Autodesk Fusion 360 part; units mm, degrees
(part 3 of 8)
  spline S13 degree 5 poles (-0.7278, 10.3745) (-0.7298, 10.3716) (-0.7338, 10.3659) (-0.7399, 10.3573) (-0.7479, 10.3459) (-0.7578, 10.3316) (-0.7677, 10.3173) (-0.7776, 10.303) (-0.7874, 10.2887) (-0.7971, 10.2744) (-0.8067, 10.2601) (-0.8163, 10.2458) (-0.8259, 10.2316) (-0.8354, 10.2173) (-0.8448, 10.203) (-0.8542, 10.1888) (-0.8635, 10.1745) (-0.8727, 10.1603) (-0.8819, 10.1461) (-0.891, 10.1318) (-0.9001, 10.1176) (-0.9091, 10.1034) (-0.918, 10.0892) (-0.9269, 10.075) (-0.9357, 10.0608) (-0.9445, 10.0467) (-0.9532, 10.0325) (-0.9619, 10.0184) (-0.9705, 10.0042) (-0.979, 9.9901) (-0.9875, 9.976) (-0.9959, 9.9619) (-1.0042, 9.9478) (-1.0125, 9.9337) (-1.0207, 9.9196) (-1.0289, 9.9056) (-1.037, 9.8915) (-1.0451, 9.8775) (-1.0531, 9.8635) (-1.061, 9.8494) (-1.0689, 9.8355) (-1.0767, 9.8215) (-1.0845, 9.8075) (-1.0922, 9.7936) (-1.0998, 9.7796) (-1.1074, 9.7657) (-1.1149, 9.7518) (-1.1224, 9.7379) (-1.1298, 9.7241) (-1.1371, 9.7102) (-1.1444, 9.6964) (-1.1516, 9.6825) (-1.1588, 9.6687) (-1.1659, 9.655) (-1.1729, 9.6412) (-1.1799, 9.6275) (-1.1868, 9.6137) (-1.1937, 9.6) (-1.2005, 9.5863) (-1.2073, 9.5727) (-1.214, 9.559) (-1.2206, 9.5454) (-1.2272, 9.5318) (-1.2337, 9.5182) (-1.2401, 9.5047) (-1.2465, 9.4911) (-1.2529, 9.4776) (-1.2592, 9.4641) (-1.2654, 9.4507) (-1.2716, 9.4372) (-1.2777, 9.4238) (-1.2837, 9.4104) (-1.2897, 9.397) (-1.2957, 9.3837) (-1.3015, 9.3704) (-1.3074, 9.3571) (-1.3131, 9.3438) (-1.3188, 9.3305) (-1.3245, 9.3173) (-1.3301, 9.3041) (-1.3356, 9.291) (-1.3411, 9.2778) (-1.3465, 9.2647) (-1.3518, 9.2517) (-1.3571, 9.2386) (-1.3624, 9.2256) (-1.3676, 9.2126) (-1.3727, 9.1997) (-1.3778, 9.1867) (-1.3828, 9.1738) (-1.3877, 9.161) (-1.3927, 9.1481) (-1.3975, 9.1353) (-1.4023, 9.1226) (-1.407, 9.1098) (-1.4117, 9.0971) (-1.4163, 9.0845) (-1.4209, 9.0718) (-1.4254, 9.0593) (-1.4299, 9.0467) (-1.4343, 9.0342) (-1.4386, 9.0217) (-1.4429, 9.0092) (-1.4471, 8.9968) (-1.4513, 8.9844) (-1.4554, 8.9721) (-1.4595, 8.9598) (-1.4635, 8.9475) (-1.4675, 8.9353) (-1.4714, 8.9231) (-1.4752, 8.9109) (-1.479, 8.8988) (-1.4828, 8.8868) (-1.4865, 8.8747) (-1.4901, 8.8628) (-1.4937, 8.8508) (-1.4972, 8.8389) (-1.5007, 8.8271) (-1.5041, 8.8153) (-1.5075, 8.8035) (-1.5108, 8.7918) (-1.514, 8.7801) (-1.5173, 8.7684) (-1.5204, 8.7569) (-1.5235, 8.7453) (-1.5266, 8.7338) (-1.5296, 8.7224) (-1.5325, 8.711) (-1.5354, 8.6996) (-1.5383, 8.6883) (-1.5411, 8.6771) (-1.5438, 8.6659) (-1.5465, 8.6547) (-1.5492, 8.6436) (-1.5517, 8.6325) (-1.5543, 8.6215) (-1.5568, 8.6106) (-1.5592, 8.5997) (-1.5616, 8.5889) (-1.564, 8.5781) (-1.5663, 8.5673) (-1.5685, 8.5567) (-1.5707, 8.546) (-1.5729, 8.5355) (-1.575, 8.525) (-1.577, 8.5145) (-1.5791, 8.5041) (-1.581, 8.4938) (-1.5829, 8.4835) (-1.5848, 8.4733) (-1.5866, 8.4631) (-1.5884, 8.453) (-1.5901, 8.443) (-1.5918, 8.433) (-1.5935, 8.4231) (-1.5951, 8.4132) (-1.5966, 8.4035) (-1.5981, 8.3937) (-1.5996, 8.3841) (-1.601, 8.3745) (-1.6024, 8.365) (-1.6037, 8.3555) (-1.605, 8.3461) (-1.6062, 8.3368) (-1.6074, 8.3276) (-1.6086, 8.3184) (-1.6097, 8.3093) (-1.6108, 8.3002) (-1.6118, 8.2913) (-1.6128, 8.2824) (-1.6138, 8.2735) (-1.6147, 8.2648) (-1.6156, 8.2561) (-1.6164, 8.2475) (-1.6172, 8.239) (-1.618, 8.2306) (-1.6187, 8.2222) (-1.6194, 8.2139) (-1.6201, 8.2057) (-1.6207, 8.1976) (-1.6213, 8.1895) (-1.6218, 8.1815) (-1.6223, 8.1737) (-1.6228, 8.1658) (-1.6233, 8.1581) (-1.6237, 8.1505) (-1.6241, 8.143) (-1.6244, 8.1355) (-1.6247, 8.1281) (-1.625, 8.1208) (-1.6253, 8.1136) (-1.6255, 8.1065) (-1.6257, 8.0995) (-1.6258, 8.0926) (-1.626, 8.0858) (-1.6261, 8.079) (-1.6262, 8.0724) (-1.6262, 8.0659) (-1.6263, 8.0594) (-1.6263, 8.0531) (-1.6262, 8.0468) (-1.6262, 8.0407) (-1.6261, 8.0346) (-1.626, 8.0287) (-1.6259, 8.0229) (-1.6258, 8.0171) (-1.6257, 8.0115) (-1.6255, 8.006) (-1.6253, 8.0006) (-1.6251, 7.9953) (-1.6249, 7.9901) (-1.6246, 7.985) (-1.6244, 7.9801) (-1.6241, 7.9752) (-1.6238, 7.9705) (-1.6235, 7.9659) (-1.6232, 7.9614) (-1.6229, 7.957) (-1.6226, 7.9528) (-1.6223, 7.9487) (-1.6219, 7.9447) (-1.6216, 7.9408) (-1.6212, 7.9371) (-1.6209, 7.9334) (-1.6205, 7.93) (-1.6202, 7.9266) (-1.6198, 7.9234) (-1.6195, 7.9204) (-1.6191, 7.9174) (-1.6188, 7.9146) (-1.6184, 7.912) (-1.6181, 7.9095) (-1.6178, 7.9072) (-1.6175, 7.905) (-1.6172, 7.9029) (-1.6169, 7.9011) (-1.6166, 7.8993) (-1.6164, 7.8978) (-1.6161, 7.8964) (-1.6159, 7.8951) (-1.6157, 7.8941) (-1.6156, 7.8933) (-1.6155, 7.8929) (-1.6155, 7.8926) (-1.6154, 7.8925) knots -1 -1 -1 -1 -1 -1 -0.99583333 -0.99166667 -0.9875 -0.98333333 -0.97916667 -0.975 -0.97083333 -0.96666667 -0.9625 -0.95833333 -0.95416667 -0.95 -0.94583333 -0.94166667 -0.9375 -0.93333333 -0.92916667 -0.925 -0.92083333 -0.91666667 -0.9125 -0.90833333 -0.90416667 -0.9 -0.89583333 -0.89166667 -0.8875 -0.88333333 -0.87916667 -0.875 -0.87083333 -0.86666667 -0.8625 -0.85833333 -0.85416667 -0.85 -0.84583333 -0.84166667 -0.8375 -0.83333333 -0.82916667 -0.825 -0.82083333 -0.81666667 -0.8125 -0.80833333 -0.80416667 -0.8 -0.79583333 -0.79166667 -0.7875 -0.78333333 -0.77916667 -0.775 -0.77083333 -0.76666667 -0.7625 -0.75833333 -0.75416667 -0.75 -0.74583333 -0.74166667 -0.7375 -0.73333333 -0.72916667 -0.725 -0.72083333 -0.71666667 -0.7125 -0.70833333 -0.70416667 -0.7 -0.69583333 -0.69166667 -0.6875 -0.68333333 -0.67916667 -0.675 -0.67083333 -0.66666667 -0.6625 -0.65833333 -0.65416667 -0.65 -0.64583333 -0.64166667 -0.6375 -0.63333333 -0.62916667 -0.625 -0.62083333 -0.61666667 -0.6125 -0.60833333 -0.60416667 -0.6 -0.59583333 -0.59166667 -0.5875 -0.58333333 -0.57916667 -0.575 -0.57083333 -0.56666667 -0.5625 -0.55833333 -0.55416667 -0.55 -0.54583333 -0.54166667 -0.5375 -0.53333333 -0.52916667 -0.525 -0.52083333 -0.51666667 -0.5125 -0.50833333 -0.50416667 -0.5 -0.49583333 -0.49166667 -0.4875 -0.48333333 -0.47916667 -0.475 -0.47083333 -0.46666667 -0.4625 -0.45833333 -0.45416667 -0.45 -0.44583333 -0.44166667 -0.4375 -0.43333333 -0.42916667 -0.425 -0.42083333 -0.41666667 -0.4125 -0.40833333 -0.40416667 -0.4 -0.39583333 -0.39166667 -0.3875 -0.38333333 -0.37916667 -0.375 -0.37083333 -0.36666667 -0.3625 -0.35833333 -0.35416667 -0.35 -0.34583333 -0.34166667 -0.3375 -0.33333333 -0.32916667 -0.325 -0.32083333 -0.31666667 -0.3125 -0.30833333 -0.30416667 -0.3 -0.29583333 -0.29166667 -0.2875 -0.28333333 -0.27916667 -0.275 -0.27083333 -0.26666667 -0.2625 -0.25833333 -0.25416667 -0.25 -0.24583333 -0.24166667 -0.2375 -0.23333333 -0.22916667 -0.225 -0.22083333 -0.21666667 -0.2125 -0.20833333 -0.20416667 -0.2 -0.19583333 -0.19166667 -0.1875 -0.18333333 -0.17916667 -0.175 -0.17083333 -0.16666667 -0.1625 -0.15833333 -0.15416667 -0.15 -0.14583333 -0.14166667 -0.1375 -0.13333333 -0.12916667 -0.125 -0.12083333 -0.11666667 -0.1125 -0.10833333 -0.10416667 -0.1 -0.09583333 -0.09166667 -0.0875 -0.08333333 -0.07916667 -0.075 -0.07083333 -0.06666667 -0.0625 -0.05833333 -0.05416667 -0.05 -0.04583333 -0.04166667 -0.0375 -0.03333333 -0.02916667 -0.025 -0.02083333 -0.01666667 -0.0125 -0.00833333 -0.00416667 0 0 0 0 0 0
  line L26 (-1.6154, 7.8925) -> (-1.6152, 7.8914)
  line L27 (-1.6152, 7.8914) -> (-1.147, 5.6038)
  arc A14 (-1.147, 5.6038) -> (-3.1514, 4.7736) centre (0, 0) ccw
  line L28 (-3.1514, 4.7736) -> (-4.4379, 6.7222)
  line L29 (-4.4379, 6.7222) -> (-4.4385, 6.7231)
  spline S14 degree 5 poles (-4.4385, 6.7231) (-4.4386, 6.7232) (-4.4388, 6.7235) (-4.439, 6.7238) (-4.4394, 6.7244) (-4.4401, 6.7253) (-4.4408, 6.7263) (-4.4416, 6.7275) (-4.4425, 6.7288) (-4.4436, 6.7302) (-4.4447, 6.7317) (-4.4459, 6.7334) (-4.4473, 6.7352) (-4.4487, 6.737) (-4.4502, 6.739) (-4.4519, 6.7411) (-4.4536, 6.7434) (-4.4554, 6.7457) (-4.4573, 6.7481) (-4.4593, 6.7506) (-4.4614, 6.7532) (-4.4637, 6.7559) (-4.466, 6.7587) (-4.4684, 6.7616) (-4.4708, 6.7646) (-4.4734, 6.7677) (-4.4761, 6.7708) (-4.4789, 6.774) (-4.4818, 6.7774) (-4.4847, 6.7807) (-4.4878, 6.7842) (-4.4909, 6.7877) (-4.4942, 6.7914) (-4.4975, 6.7951) (-4.5009, 6.7988) (-4.5044, 6.8026) (-4.508, 6.8065) (-4.5117, 6.8105) (-4.5155, 6.8145) (-4.5194, 6.8186) (-4.5233, 6.8227) (-4.5274, 6.8269) (-4.5315, 6.8312) (-4.5357, 6.8355) (-4.54, 6.8399) (-4.5444, 6.8443) (-4.5489, 6.8488) (-4.5535, 6.8533) (-4.5582, 6.8579) (-4.5629, 6.8626) (-4.5678, 6.8672) (-4.5727, 6.872) (-4.5777, 6.8768) (-4.5828, 6.8816) (-4.588, 6.8864) (-4.5932, 6.8914) (-4.5986, 6.8963) (-4.604, 6.9013) (-4.6096, 6.9063) (-4.6152, 6.9114) (-4.6208, 6.9165) (-4.6266, 6.9216) (-4.6325, 6.9268) (-4.6384, 6.932) (-4.6444, 6.9373) (-4.6505, 6.9426) (-4.6567, 6.9479) (-4.663, 6.9532) (-4.6693, 6.9586) (-4.6758, 6.964) (-4.6823, 6.9694) (-4.6889, 6.9749) (-4.6956, 6.9804) (-4.7023, 6.9859) (-4.7092, 6.9914) (-4.7161, 6.997) (-4.7231, 7.0025) (-4.7301, 7.0082) (-4.7373, 7.0138) (-4.7445, 7.0194) (-4.7518, 7.0251) (-4.7592, 7.0308) (-4.7667, 7.0365) (-4.7743, 7.0422) (-4.7819, 7.048) (-4.7896, 7.0537) (-4.7974, 7.0595) (-4.8052, 7.0653) (-4.8132, 7.0711) (-4.8212, 7.0769) (-4.8293, 7.0828) (-4.8375, 7.0886) (-4.8457, 7.0945) (-4.854, 7.1004) (-4.8624, 7.1062) (-4.8709, 7.1121) (-4.8794, 7.118) (-4.8881, 7.1239) (-4.8968, 7.1299) (-4.9055, 7.1358) (-4.9144, 7.1417) (-4.9233, 7.1477) (-4.9323, 7.1536) (-4.9414, 7.1596) (-4.9505, 7.1655) (-4.9597, 7.1715) (-4.969, 7.1775) (-4.9784, 7.1834) (-4.9878, 7.1894) (-4.9973, 7.1954) (-5.0069, 7.2014) (-5.0165, 7.2074) (-5.0262, 7.2133) (-5.036, 7.2193) (-5.0459, 7.2253) (-5.0558, 7.2313) (-5.0658, 7.2373) (-5.0759, 7.2432) (-5.0861, 7.2492) (-5.0963, 7.2552) (-5.1066, 7.2612) (-5.1169, 7.2671) (-5.1274, 7.2731) (-5.1379, 7.279) (-5.1484, 7.285) (-5.1591, 7.2909) (-5.1698, 7.2969) (-5.1805, 7.3028) (-5.1914, 7.3087) (-5.2023, 7.3147) (-5.2133, 7.3206) (-5.2243, 7.3265) (-5.2354, 7.3324) (-5.2466, 7.3383) (-5.2578, 7.3441) (-5.2692, 7.35) (-5.2805, 7.3559) (-5.292, 7.3617) (-5.3035, 7.3675) (-5.3151, 7.3734) (-5.3267, 7.3792) (-5.3384, 7.385) (-5.3502, 7.3908) (-5.362, 7.3965) (-5.3739, 7.4023) (-5.3859, 7.408) (-5.3979, 7.4138) (-5.41, 7.4195) (-5.4222, 7.4252) (-5.4344, 7.4309) (-5.4467, 7.4366) (-5.4591, 7.4422) (-5.4715, 7.4478) (-5.484, 7.4535) (-5.4965, 7.4591) (-5.5091, 7.4647) (-5.5218, 7.4702) (-5.5345, 7.4758) (-5.5473, 7.4813) (-5.5601, 7.4868) (-5.5731, 7.4923) (-5.586, 7.4978) (-5.5991, 7.5033) (-5.6122, 7.5087) (-5.6253, 7.5141) (-5.6385, 7.5195) (-5.6518, 7.5249) (-5.6651, 7.5302) (-5.6785, 7.5356) (-5.692, 7.5409) (-5.7055, 7.5462) (-5.7191, 7.5514) (-5.7327, 7.5567) (-5.7464, 7.5619) (-5.7602, 7.5671) (-5.774, 7.5722) (-5.7878, 7.5774) (-5.8018, 7.5825) (-5.8158, 7.5876) (-5.8298, 7.5927) (-5.8439, 7.5977) (-5.8581, 7.6028) (-5.8723, 7.6077) (-5.8865, 7.6127) (-5.9009, 7.6177) (-5.9152, 7.6226) (-5.9297, 7.6275) (-5.9442, 7.6323) (-5.9587, 7.6372) (-5.9733, 7.642) (-5.988, 7.6467) (-6.0027, 7.6515) (-6.0175, 7.6562) (-6.0323, 7.6609) (-6.0472, 7.6656) (-6.0621, 7.6702) (-6.0771, 7.6748) (-6.0921, 7.6794) (-6.1072, 7.6839) (-6.1224, 7.6884) (-6.1376, 7.6929) (-6.1528, 7.6974) (-6.1681, 7.7018) (-6.1835, 7.7062) (-6.1989, 7.7105) (-6.2144, 7.7149) (-6.2299, 7.7192) (-6.2454, 7.7234) (-6.2611, 7.7276) (-6.2767, 7.7318) (-6.2925, 7.736) (-6.3082, 7.7401) (-6.324, 7.7442) (-6.3399, 7.7483) (-6.3558, 7.7523) (-6.3718, 7.7563) (-6.3878, 7.7603) (-6.4039, 7.7642) (-6.42, 7.7681) (-6.4362, 7.7719) (-6.4524, 7.7758) (-6.4687, 7.7796) (-6.485, 7.7833) (-6.5014, 7.787) (-6.5178, 7.7907) (-6.5343, 7.7943) (-6.5508, 7.7979) (-6.5673, 7.8015) (-6.5839, 7.805) (-6.6006, 7.8085) (-6.6173, 7.812) (-6.634, 7.8154) (-6.6508, 7.8188) (-6.6677, 7.8221) (-6.6845, 7.8254) (-6.7015, 7.8287) (-6.7185, 7.8319) (-6.7355, 7.8351) (-6.7525, 7.8383) (-6.7697, 7.8414) (-6.7868, 7.8445) (-6.8006, 7.8469) (-6.8109, 7.8487) (-6.8178, 7.8499) (-6.8213, 7.8505) knots 0 0 0 0 0 0 0.00416667 0.00833333 0.0125 0.01666667 0.02083333 0.025 0.02916667 0.03333333 0.0375 0.04166667 0.04583333 0.05 0.05416667 0.05833333 0.0625 0.06666667 0.07083333 0.075 0.07916667 0.08333333 0.0875 0.09166667 0.09583333 0.1 0.10416667 0.10833333 0.1125 0.11666667 0.12083333 0.125 0.12916667 0.13333333 0.1375 0.14166667 0.14583333 0.15 0.15416667 0.15833333 0.1625 0.16666667 0.17083333 0.175 0.17916667 0.18333333 0.1875 0.19166667 0.19583333 0.2 0.20416667 0.20833333 0.2125 0.21666667 0.22083333 0.225 0.22916667 0.23333333 0.2375 0.24166667 0.24583333 0.25 0.25416667 0.25833333 0.2625 0.26666667 0.27083333 0.275 0.27916667 0.28333333 0.2875 0.29166667 0.29583333 0.3 0.30416667 0.30833333 0.3125 0.31666667 0.32083333 0.325 0.32916667 0.33333333 0.3375 0.34166667 0.34583333 0.35 0.35416667 0.35833333 0.3625 0.36666667 0.37083333 0.375 0.37916667 0.38333333 0.3875 0.39166667 0.39583333 0.4 0.40416667 0.40833333 0.4125 0.41666667 0.42083333 0.425 0.42916667 0.43333333 0.4375 0.44166667 0.44583333 0.45 0.45416667 0.45833333 0.4625 0.46666667 0.47083333 0.475 0.47916667 0.48333333 0.4875 0.49166667 0.49583333 0.5 0.50416667 0.50833333 0.5125 0.51666667 0.52083333 0.525 0.52916667 0.53333333 0.5375 0.54166667 0.54583333 0.55 0.55416667 0.55833333 0.5625 0.56666667 0.57083333 0.575 0.57916667 0.58333333 0.5875 0.59166667 0.59583333 0.6 0.60416667 0.60833333 0.6125 0.61666667 0.62083333 0.625 0.62916667 0.63333333 0.6375 0.64166667 0.64583333 0.65 0.65416667 0.65833333 0.6625 0.66666667 0.67083333 0.675 0.67916667 0.68333333 0.6875 0.69166667 0.69583333 0.7 0.70416667 0.70833333 0.7125 0.71666667 0.72083333 0.725 0.72916667 0.73333333 0.7375 0.74166667 0.74583333 0.75 0.75416667 0.75833333 0.7625 0.76666667 0.77083333 0.775 0.77916667 0.78333333 0.7875 0.79166667 0.79583333 0.8 0.80416667 0.80833333 0.8125 0.81666667 0.82083333 0.825 0.82916667 0.83333333 0.8375 0.84166667 0.84583333 0.85 0.85416667 0.85833333 0.8625 0.86666667 0.87083333 0.875 0.87916667 0.88333333 0.8875 0.89166667 0.89583333 0.9 0.90416667 0.90833333 0.9125 0.91666667 0.92083333 0.925 0.92916667 0.93333333 0.9375 0.94166667 0.94583333 0.95 0.95416667 0.95833333 0.9625 0.96666667 0.97083333 0.975 0.97916667 0.98333333 0.9875 0.99166667 0.99583333 1 1 1 1 1 1
  arc A15 (-6.8213, 7.8505) -> (-7.8505, 6.8213) centre (0, 0) ccw
  spline S15 degree 5 poles (-7.8505, 6.8213) (-7.8499, 6.8178) (-7.8487, 6.8109) (-7.8469, 6.8006) (-7.8445, 6.7868) (-7.8414, 6.7697) (-7.8383, 6.7525) (-7.8351, 6.7355) (-7.8319, 6.7185) (-7.8287, 6.7015) (-7.8254, 6.6845) (-7.8221, 6.6677) (-7.8188, 6.6508) (-7.8154, 6.634) (-7.812, 6.6173) (-7.8085, 6.6006) (-7.805, 6.5839) (-7.8015, 6.5673) (-7.7979, 6.5508) (-7.7943, 6.5343) (-7.7907, 6.5178) (-7.787, 6.5014) (-7.7833, 6.485) (-7.7796, 6.4687) (-7.7758, 6.4524) (-7.7719, 6.4362) (-7.7681, 6.42) (-7.7642, 6.4039) (-7.7603, 6.3878) (-7.7563, 6.3718) (-7.7523, 6.3558) (-7.7483, 6.3399) (-7.7442, 6.324) (-7.7401, 6.3082) (-7.736, 6.2925) (-7.7318, 6.2767) (-7.7276, 6.2611) (-7.7234, 6.2454) (-7.7192, 6.2299) (-7.7149, 6.2144) (-7.7105, 6.1989) (-7.7062, 6.1835) (-7.7018, 6.1681) (-7.6974, 6.1528) (-7.6929, 6.1376) (-7.6884, 6.1224) (-7.6839, 6.1072) (-7.6794, 6.0921) (-7.6748, 6.0771) (-7.6702, 6.0621) (-7.6656, 6.0472) (-7.6609, 6.0323) (-7.6562, 6.0175) (-7.6515, 6.0027) (-7.6467, 5.988) (-7.642, 5.9733) (-7.6372, 5.9587) (-7.6323, 5.9442) (-7.6275, 5.9297) (-7.6226, 5.9152) (-7.6177, 5.9009) (-7.6127, 5.8865) (-7.6077, 5.8723) (-7.6028, 5.8581) (-7.5977, 5.8439) (-7.5927, 5.8298) (-7.5876, 5.8158) (-7.5825, 5.8018) (-7.5774, 5.7878) (-7.5722, 5.774) (-7.5671, 5.7602) (-7.5619, 5.7464) (-7.5567, 5.7327) (-7.5514, 5.7191) (-7.5462, 5.7055) (-7.5409, 5.692) (-7.5356, 5.6785) (-7.5302, 5.6651) (-7.5249, 5.6518) (-7.5195, 5.6385) (-7.5141, 5.6253) (-7.5087, 5.6122) (-7.5033, 5.5991) (-7.4978, 5.586) (-7.4923, 5.5731) (-7.4868, 5.5601) (-7.4813, 5.5473) (-7.4758, 5.5345) (-7.4702, 5.5218) (-7.4647, 5.5091) (-7.4591, 5.4965) (-7.4535, 5.484) (-7.4478, 5.4715) (-7.4422, 5.4591) (-7.4366, 5.4467) (-7.4309, 5.4344) (-7.4252, 5.4222) (-7.4195, 5.41) (-7.4138, 5.3979) (-7.408, 5.3859) (-7.4023, 5.3739) (-7.3965, 5.362) (-7.3908, 5.3502) (-7.385, 5.3384) (-7.3792, 5.3267) (-7.3734, 5.3151) (-7.3675, 5.3035) (-7.3617, 5.292) (-7.3559, 5.2805) (-7.35, 5.2692) (-7.3441, 5.2578) (-7.3383, 5.2466) (-7.3324, 5.2354) (-7.3265, 5.2243) (-7.3206, 5.2133) (-7.3147, 5.2023) (-7.3087, 5.1914) (-7.3028, 5.1805) (-7.2969, 5.1698) (-7.2909, 5.1591) (-7.285, 5.1484) (-7.279, 5.1379) (-7.2731, 5.1274) (-7.2671, 5.1169) (-7.2612, 5.1066) (-7.2552, 5.0963) (-7.2492, 5.0861) (-7.2432, 5.0759) (-7.2373, 5.0658) (-7.2313, 5.0558) (-7.2253, 5.0459) (-7.2193, 5.036) (-7.2133, 5.0262) (-7.2074, 5.0165) (-7.2014, 5.0069) (-7.1954, 4.9973) (-7.1894, 4.9878) (-7.1834, 4.9784) (-7.1775, 4.969) (-7.1715, 4.9597) (-7.1655, 4.9505) (-7.1596, 4.9414) (-7.1536, 4.9323) (-7.1477, 4.9233) (-7.1417, 4.9144) (-7.1358, 4.9055) (-7.1299, 4.8968) (-7.1239, 4.8881) (-7.118, 4.8794) (-7.1121, 4.8709) (-7.1062, 4.8624) (-7.1004, 4.854) (-7.0945, 4.8457) (-7.0886, 4.8375) (-7.0828, 4.8293) (-7.0769, 4.8212) (-7.0711, 4.8132) (-7.0653, 4.8052) (-7.0595, 4.7974) (-7.0537, 4.7896) (-7.048, 4.7819) (-7.0422, 4.7743) (-7.0365, 4.7667) (-7.0308, 4.7592) (-7.0251, 4.7518) (-7.0194, 4.7445) (-7.0138, 4.7373) (-7.0082, 4.7301) (-7.0025, 4.7231) (-6.997, 4.7161) (-6.9914, 4.7092) (-6.9859, 4.7023) (-6.9804, 4.6956) (-6.9749, 4.6889) (-6.9694, 4.6823) (-6.964, 4.6758) (-6.9586, 4.6693) (-6.9532, 4.663) (-6.9479, 4.6567) (-6.9426, 4.6505) (-6.9373, 4.6444) (-6.932, 4.6384) (-6.9268, 4.6325) (-6.9216, 4.6266) (-6.9165, 4.6208) (-6.9114, 4.6152) (-6.9063, 4.6096) (-6.9013, 4.604) (-6.8963, 4.5986) (-6.8914, 4.5932) (-6.8864, 4.588) (-6.8816, 4.5828) (-6.8768, 4.5777) (-6.872, 4.5727) (-6.8672, 4.5678) (-6.8626, 4.5629) (-6.8579, 4.5582) (-6.8533, 4.5535) (-6.8488, 4.5489) (-6.8443, 4.5444) (-6.8399, 4.54) (-6.8355, 4.5357) (-6.8312, 4.5315) (-6.8269, 4.5274) (-6.8227, 4.5233) (-6.8186, 4.5194) (-6.8145, 4.5155) (-6.8105, 4.5117) (-6.8065, 4.508) (-6.8026, 4.5044) (-6.7988, 4.5009) (-6.7951, 4.4975) (-6.7914, 4.4942) (-6.7877, 4.4909) (-6.7842, 4.4878) (-6.7807, 4.4847) (-6.7774, 4.4818) (-6.774, 4.4789) (-6.7708, 4.4761) (-6.7677, 4.4734) (-6.7646, 4.4708) (-6.7616, 4.4684) (-6.7587, 4.466) (-6.7559, 4.4637) (-6.7532, 4.4614) (-6.7506, 4.4593) (-6.7481, 4.4573) (-6.7457, 4.4554) (-6.7434, 4.4536) (-6.7411, 4.4519) (-6.739, 4.4502) (-6.737, 4.4487) (-6.7352, 4.4473) (-6.7334, 4.4459) (-6.7317, 4.4447) (-6.7302, 4.4436) (-6.7288, 4.4425) (-6.7275, 4.4416) (-6.7263, 4.4408) (-6.7253, 4.4401) (-6.7244, 4.4394) (-6.7238, 4.439) (-6.7235, 4.4388) (-6.7232, 4.4386) (-6.7231, 4.4385) knots -1 -1 -1 -1 -1 -1 -0.99583333 -0.99166667 -0.9875 -0.98333333 -0.97916667 -0.975 -0.97083333 -0.96666667 -0.9625 -0.95833333 -0.95416667 -0.95 -0.94583333 -0.94166667 -0.9375 -0.93333333 -0.92916667 -0.925 -0.92083333 -0.91666667 -0.9125 -0.90833333 -0.90416667 -0.9 -0.89583333 -0.89166667 -0.8875 -0.88333333 -0.87916667 -0.875 -0.87083333 -0.86666667 -0.8625 -0.85833333 -0.85416667 -0.85 -0.84583333 -0.84166667 -0.8375 -0.83333333 -0.82916667 -0.825 -0.82083333 -0.81666667 -0.8125 -0.80833333 -0.80416667 -0.8 -0.79583333 -0.79166667 -0.7875 -0.78333333 -0.77916667 -0.775 -0.77083333 -0.76666667 -0.7625 -0.75833333 -0.75416667 -0.75 -0.74583333 -0.74166667 -0.7375 -0.73333333 -0.72916667 -0.725 -0.72083333 -0.71666667 -0.7125 -0.70833333 -0.70416667 -0.7 -0.69583333 -0.69166667 -0.6875 -0.68333333 -0.67916667 -0.675 -0.67083333 -0.66666667 -0.6625 -0.65833333 -0.65416667 -0.65 -0.64583333 -0.64166667 -0.6375 -0.63333333 -0.62916667 -0.625 -0.62083333 -0.61666667 -0.6125 -0.60833333 -0.60416667 -0.6 -0.59583333 -0.59166667 -0.5875 -0.58333333 -0.57916667 -0.575 -0.57083333 -0.56666667 -0.5625 -0.55833333 -0.55416667 -0.55 -0.54583333 -0.54166667 -0.5375 -0.53333333 -0.52916667 -0.525 -0.52083333 -0.51666667 -0.5125 -0.50833333 -0.50416667 -0.5 -0.49583333 -0.49166667 -0.4875 -0.48333333 -0.47916667 -0.475 -0.47083333 -0.46666667 -0.4625 -0.45833333 -0.45416667 -0.45 -0.44583333 -0.44166667 -0.4375 -0.43333333 -0.42916667 -0.425 -0.42083333 -0.41666667 -0.4125 -0.40833333 -0.40416667 -0.4 -0.39583333 -0.39166667 -0.3875 -0.38333333 -0.37916667 -0.375 -0.37083333 -0.36666667 -0.3625 -0.35833333 -0.35416667 -0.35 -0.34583333 -0.34166667 -0.3375 -0.33333333 -0.32916667 -0.325 -0.32083333 -0.31666667 -0.3125 -0.30833333 -0.30416667 -0.3 -0.29583333 -0.29166667 -0.2875 -0.28333333 -0.27916667 -0.275 -0.27083333 -0.26666667 -0.2625 -0.25833333 -0.25416667 -0.25 -0.24583333 -0.24166667 -0.2375 -0.23333333 -0.22916667 -0.225 -0.22083333 -0.21666667 -0.2125 -0.20833333 -0.20416667 -0.2 -0.19583333 -0.19166667 -0.1875 -0.18333333 -0.17916667 -0.175 -0.17083333 -0.16666667 -0.1625 -0.15833333 -0.15416667 -0.15 -0.14583333 -0.14166667 -0.1375 -0.13333333 -0.12916667 -0.125 -0.12083333 -0.11666667 -0.1125 -0.10833333 -0.10416667 -0.1 -0.09583333 -0.09166667 -0.0875 -0.08333333 -0.07916667 -0.075 -0.07083333 -0.06666667 -0.0625 -0.05833333 -0.05416667 -0.05 -0.04583333 -0.04166667 -0.0375 -0.03333333 -0.02916667 -0.025 -0.02083333 -0.01666667 -0.0125 -0.00833333 -0.00416667 0 0 0 0 0 0
  line L30 (-6.7231, 4.4385) -> (-6.7222, 4.4379)
  line L31 (-6.7222, 4.4379) -> (-4.7736, 3.1514)
  circle A16 centre (0, 0) radius 2.9
  dimension "d7" = 5.8
  constraint concentric A0 A16
  measures "d7" diameter of A16
sketch "Sketch1 (2)" plane through (0, 0, 0) normal (0, 0, 1) x (1, 0, 0) in component "Component"
  spline S0 degree 5 poles (8.6134, -1.763) (8.6136, -1.763) (8.6139, -1.7631) (8.6144, -1.7632) (8.6152, -1.7633) (8.6164, -1.7635) (8.6178, -1.7638) (8.6193, -1.764) (8.6211, -1.7643) (8.6231, -1.7646) (8.6252, -1.7649) (8.6275, -1.7653) (8.6299, -1.7656) (8.6326, -1.766) (8.6354, -1.7664) (8.6383, -1.7667) (8.6414, -1.7671) (8.6447, -1.7675) (8.6482, -1.7679) (8.6518, -1.7683) (8.6555, -1.7687) (8.6594, -1.7691) (8.6634, -1.7695) (8.6676, -1.7698) (8.6719, -1.7702) (8.6764, -1.7706) (8.681, -1.7709) (8.6857, -1.7713) (8.6906, -1.7716) (8.6956, -1.772) (8.7007, -1.7723) (8.706, -1.7726) (8.7114, -1.7729) (8.7169, -1.7732) (8.7226, -1.7734) (8.7283, -1.7736) (8.7342, -1.7739) (8.7402, -1.7741) (8.7464, -1.7742) (8.7526, -1.7744) (8.759, -1.7745) (8.7655, -1.7746) (8.772, -1.7747) (8.7787, -1.7748) (8.7856, -1.7748) (8.7925, -1.7748) (8.7995, -1.7748) (8.8067, -1.7747) (8.8139, -1.7747) (8.8212, -1.7746) (8.8287, -1.7744) (8.8362, -1.7743) (8.8439, -1.7741) (8.8517, -1.7738) (8.8595, -1.7736) (8.8675, -1.7733) (8.8755, -1.7729) (8.8836, -1.7726) (8.8919, -1.7722) (8.9002, -1.7717) (8.9086, -1.7712) (8.9172, -1.7707) (8.9258, -1.7702) (8.9345, -1.7696) (8.9432, -1.769) (8.9521, -1.7683) (8.9611, -1.7676) (8.9701, -1.7669) (8.9792, -1.7661) (8.9885, -1.7653) (8.9978, -1.7644) (9.0071, -1.7635) (9.0166, -1.7625) (9.0261, -1.7615) (9.0358, -1.7605) (9.0455, -1.7594) (9.0552, -1.7583) (9.0651, -1.7571) (9.075, -1.7559) (9.0851, -1.7547) (9.0951, -1.7534) (9.1053, -1.752) (9.1155, -1.7506) (9.1258, -1.7492) (9.1362, -1.7477) (9.1467, -1.7462) (9.1572, -1.7446) (9.1678, -1.743) (9.1785, -1.7413) (9.1892, -1.7396) (9.2, -1.7378) (9.2109, -1.736) (9.2218, -1.7341) (9.2328, -1.7322) (9.2439, -1.7302) (9.255, -1.7282) (9.2662, -1.7261) (9.2774, -1.724) (9.2888, -1.7218) (9.3001, -1.7196) (9.3116, -1.7173) (9.3231, -1.7149) (9.3347, -1.7126) (9.3463, -1.7101) (9.358, -1.7076) (9.3697, -1.7051) (9.3815, -1.7025) (9.3934, -1.6998) (9.4053, -1.6971) (9.4173, -1.6944) (9.4293, -1.6916) (9.4414, -1.6887) (9.4535, -1.6858) (9.4657, -1.6828) (9.4779, -1.6798) (9.4902, -1.6767) (9.5026, -1.6736) (9.515, -1.6704) (9.5274, -1.6671) (9.5399, -1.6638) (9.5525, -1.6604) (9.5651, -1.657) (9.5777, -1.6536) (9.5904, -1.65) (9.6032, -1.6464) (9.616, -1.6428) (9.6288, -1.6391) (9.6417, -1.6353) (9.6546, -1.6315) (9.6676, -1.6276) (9.6806, -1.6237) (9.6937, -1.6197) (9.7068, -1.6156) (9.72, -1.6115) (9.7332, -1.6074) (9.7464, -1.6031) (9.7597, -1.5989) (9.773, -1.5945) (9.7864, -1.5901) (9.7998, -1.5857) (9.8132, -1.5811) (9.8267, -1.5766) (9.8403, -1.5719) (9.8538, -1.5672) (9.8674, -1.5625) (9.8811, -1.5576) (9.8948, -1.5528) (9.9085, -1.5478) (9.9222, -1.5428) (9.936, -1.5378) (9.9498, -1.5326) (9.9637, -1.5275) (9.9776, -1.5222) (9.9915, -1.5169) (10.0055, -1.5116) (10.0195, -1.5061) (10.0335, -1.5007) (10.0476, -1.4951) (10.0617, -1.4895) (10.0758, -1.4838) (10.0899, -1.4781) (10.1041, -1.4723) (10.1183, -1.4665) (10.1326, -1.4605) (10.1469, -1.4546) (10.1612, -1.4485) (10.1755, -1.4424) (10.1899, -1.4363) (10.2043, -1.43) (10.2187, -1.4238) (10.2331, -1.4174) (10.2476, -1.411) (10.2621, -1.4045) (10.2767, -1.398) (10.2912, -1.3914) (10.3058, -1.3847) (10.3204, -1.378) (10.335, -1.3712) (10.3497, -1.3644) (10.3644, -1.3575) (10.3791, -1.3505) (10.3938, -1.3435) (10.4085, -1.3364) (10.4233, -1.3292) (10.4381, -1.322) (10.4529, -1.3147) (10.4677, -1.3073) (10.4826, -1.2999) (10.4975, -1.2924) (10.5124, -1.2849) (10.5273, -1.2773) (10.5422, -1.2696) (10.5572, -1.2619) (10.5722, -1.2541) (10.5872, -1.2463) (10.6022, -1.2383) (10.6172, -1.2303) (10.6322, -1.2223) (10.6473, -1.2142) (10.6624, -1.206) (10.6775, -1.1978) (10.6926, -1.1895) (10.7077, -1.1811) (10.7229, -1.1727) (10.738, -1.1642) (10.7532, -1.1556) (10.7684, -1.147) (10.7836, -1.1383) (10.7988, -1.1296) (10.8141, -1.1208) (10.8293, -1.1119) (10.8446, -1.103) (10.8598, -1.094) (10.8751, -1.0849) (10.8904, -1.0758) (10.9057, -1.0666) (10.921, -1.0573) (10.9364, -1.048) (10.9517, -1.0386) (10.967, -1.0292) (10.9824, -1.0197) (10.9978, -1.0101) (11.0131, -1.0004) (11.0285, -0.9907) (11.0439, -0.981) (11.0593, -0.9711) (11.0747, -0.9612) (11.0902, -0.9513) (11.1056, -0.9413) (11.121, -0.9312) (11.1365, -0.921) (11.1519, -0.9108) (11.1674, -0.9005) (11.1828, -0.8902) (11.1983, -0.8798) (11.2138, -0.8693) (11.2292, -0.8588) (11.2447, -0.8482) (11.2602, -0.8375) (11.2757, -0.8268) (11.2912, -0.816) (11.3036, -0.8073) (11.3129, -0.8008) (11.3191, -0.7964) (11.3222, -0.7942) knots 0 0 0 0 0 0 0.00416667 0.00833333 0.0125 0.01666667 0.02083333 0.025 0.02916667 0.03333333 0.0375 0.04166667 0.04583333 0.05 0.05416667 0.05833333 0.0625 0.06666667 0.07083333 0.075 0.07916667 0.08333333 0.0875 0.09166667 0.09583333 0.1 0.10416667 0.10833333 0.1125 0.11666667 0.12083333 0.125 0.12916667 0.13333333 0.1375 0.14166667 0.14583333 0.15 0.15416667 0.15833333 0.1625 0.16666667 0.17083333 0.175 0.17916667 0.18333333 0.1875 0.19166667 0.19583333 0.2 0.20416667 0.20833333 0.2125 0.21666667 0.22083333 0.225 0.22916667 0.23333333 0.2375 0.24166667 0.24583333 0.25 0.25416667 0.25833333 0.2625 0.26666667 0.27083333 0.275 0.27916667 0.28333333 0.2875 0.29166667 0.29583333 0.3 0.30416667 0.30833333 0.3125 0.31666667 0.32083333 0.325 0.32916667 0.33333333 0.3375 0.34166667 0.34583333 0.35 0.35416667 0.35833333 0.3625 0.36666667 0.37083333 0.375 0.37916667 0.38333333 0.3875 0.39166667 0.39583333 0.4 0.40416667 0.40833333 0.4125 0.41666667 0.42083333 0.425 0.42916667 0.43333333 0.4375 0.44166667 0.44583333 0.45 0.45416667 0.45833333 0.4625 0.46666667 0.47083333 0.475 0.47916667 0.48333333 0.4875 0.49166667 0.49583333 0.5 0.50416667 0.50833333 0.5125 0.51666667 0.52083333 0.525 0.52916667 0.53333333 0.5375 0.54166667 0.54583333 0.55 0.55416667 0.55833333 0.5625 0.56666667 0.57083333 0.575 0.57916667 0.58333333 0.5875 0.59166667 0.59583333 0.6 0.60416667 0.60833333 0.6125 0.61666667 0.62083333 0.625 0.62916667 0.63333333 0.6375 0.64166667 0.64583333 0.65 0.65416667 0.65833333 0.6625 0.66666667 0.67083333 0.675 0.67916667 0.68333333 0.6875 0.69166667 0.69583333 0.7 0.70416667 0.70833333 0.7125 0.71666667 0.72083333 0.725 0.72916667 0.73333333 0.7375 0.74166667 0.74583333 0.75 0.75416667 0.75833333 0.7625 0.76666667 0.77083333 0.775 0.77916667 0.78333333 0.7875 0.79166667 0.79583333 0.8 0.80416667 0.80833333 0.8125 0.81666667 0.82083333 0.825 0.82916667 0.83333333 0.8375 0.84166667 0.84583333 0.85 0.85416667 0.85833333 0.8625 0.86666667 0.87083333 0.875 0.87916667 0.88333333 0.8875 0.89166667 0.89583333 0.9 0.90416667 0.90833333 0.9125 0.91666667 0.92083333 0.925 0.92916667 0.93333333 0.9375 0.94166667 0.94583333 0.95 0.95416667 0.95833333 0.9625 0.96666667 0.97083333 0.975 0.97916667 0.98333333 0.9875 0.99166667 0.99583333 1 1 1 1 1 1
  spline S1 degree 5 poles (8.6134, 1.763) (8.6136, 1.763) (8.6139, 1.7631) (8.6144, 1.7632) (8.6152, 1.7633) (8.6164, 1.7635) (8.6178, 1.7638) (8.6193, 1.764) (8.6211, 1.7643) (8.6231, 1.7646) (8.6252, 1.7649) (8.6275, 1.7653) (8.6299, 1.7656) (8.6326, 1.766) (8.6354, 1.7664) (8.6383, 1.7667) (8.6414, 1.7671) (8.6447, 1.7675) (8.6482, 1.7679) (8.6518, 1.7683) (8.6555, 1.7687) (8.6594, 1.7691) (8.6634, 1.7695) (8.6676, 1.7698) (8.6719, 1.7702) (8.6764, 1.7706) (8.681, 1.7709) (8.6857, 1.7713) (8.6906, 1.7716) (8.6956, 1.772) (8.7007, 1.7723) (8.706, 1.7726) (8.7114, 1.7729) (8.7169, 1.7732) (8.7226, 1.7734) (8.7283, 1.7736) (8.7342, 1.7739) (8.7402, 1.7741) (8.7464, 1.7742) (8.7526, 1.7744) (8.759, 1.7745) (8.7655, 1.7746) (8.772, 1.7747) (8.7787, 1.7748) (8.7856, 1.7748) (8.7925, 1.7748) (8.7995, 1.7748) (8.8067, 1.7747) (8.8139, 1.7747) (8.8212, 1.7746) (8.8287, 1.7744) (8.8362, 1.7743) (8.8439, 1.7741) (8.8517, 1.7738) (8.8595, 1.7736) (8.8675, 1.7733) (8.8755, 1.7729) (8.8836, 1.7726) (8.8919, 1.7722) (8.9002, 1.7717) (8.9086, 1.7712) (8.9172, 1.7707) (8.9258, 1.7702) (8.9345, 1.7696) (8.9432, 1.769) (8.9521, 1.7683) (8.9611, 1.7676) (8.9701, 1.7669) (8.9792, 1.7661) (8.9885, 1.7653) (8.9978, 1.7644) (9.0071, 1.7635) (9.0166, 1.7625) (9.0261, 1.7615) (9.0358, 1.7605) (9.0455, 1.7594) (9.0552, 1.7583) (9.0651, 1.7571) (9.075, 1.7559) (9.0851, 1.7547) (9.0951, 1.7534) (9.1053, 1.752) (9.1155, 1.7506) (9.1258, 1.7492) (9.1362, 1.7477) (9.1467, 1.7462) (9.1572, 1.7446) (9.1678, 1.743) (9.1785, 1.7413) (9.1892, 1.7396) (9.2, 1.7378) (9.2109, 1.736) (9.2218, 1.7341) (9.2328, 1.7322) (9.2439, 1.7302) (9.255, 1.7282) (9.2662, 1.7261) (9.2774, 1.724) (9.2888, 1.7218) (9.3001, 1.7196) (9.3116, 1.7173) (9.3231, 1.7149) (9.3347, 1.7126) (9.3463, 1.7101) (9.358, 1.7076) (9.3697, 1.7051) (9.3815, 1.7025) (9.3934, 1.6998) (9.4053, 1.6971) (9.4173, 1.6944) (9.4293, 1.6916) (9.4414, 1.6887) (9.4535, 1.6858) (9.4657, 1.6828) (9.4779, 1.6798) (9.4902, 1.6767) (9.5026, 1.6736) (9.515, 1.6704) (9.5274, 1.6671) (9.5399, 1.6638) (9.5525, 1.6604) (9.5651, 1.657) (9.5777, 1.6536) (9.5904, 1.65) (9.6032, 1.6464) (9.616, 1.6428) (9.6288, 1.6391) (9.6417, 1.6353) (9.6546, 1.6315) (9.6676, 1.6276) (9.6806, 1.6237) (9.6937, 1.6197) (9.7068, 1.6156) (9.72, 1.6115) (9.7332, 1.6074) (9.7464, 1.6031) (9.7597, 1.5989) (9.773, 1.5945) (9.7864, 1.5901) (9.7998, 1.5857) (9.8132, 1.5811) (9.8267, 1.5766) (9.8403, 1.5719) (9.8538, 1.5672) (9.8674, 1.5625) (9.8811, 1.5576) (9.8948, 1.5528) (9.9085, 1.5478) (9.9222, 1.5428) (9.936, 1.5378) (9.9498, 1.5326) (9.9637, 1.5275) (9.9776, 1.5222) (9.9915, 1.5169) (10.0055, 1.5116) (10.0195, 1.5061) (10.0335, 1.5007) (10.0476, 1.4951) (10.0617, 1.4895) (10.0758, 1.4838) (10.0899, 1.4781) (10.1041, 1.4723) (10.1183, 1.4665) (10.1326, 1.4605) (10.1469, 1.4546) (10.1612, 1.4485) (10.1755, 1.4424) (10.1899, 1.4363) (10.2043, 1.43) (10.2187, 1.4238) (10.2331, 1.4174) (10.2476, 1.411) (10.2621, 1.4045) (10.2767, 1.398) (10.2912, 1.3914) (10.3058, 1.3847) (10.3204, 1.378) (10.335, 1.3712) (10.3497, 1.3644) (10.3644, 1.3575) (10.3791, 1.3505) (10.3938, 1.3435) (10.4085, 1.3364) (10.4233, 1.3292) (10.4381, 1.322) (10.4529, 1.3147) (10.4677, 1.3073) (10.4826, 1.2999) (10.4975, 1.2924) (10.5124, 1.2849) (10.5273, 1.2773) (10.5422, 1.2696) (10.5572, 1.2619) (10.5722, 1.2541) (10.5872, 1.2463) (10.6022, 1.2383) (10.6172, 1.2303) (10.6322, 1.2223) (10.6473, 1.2142) (10.6624, 1.206) (10.6775, 1.1978) (10.6926, 1.1895) (10.7077, 1.1811) (10.7229, 1.1727) (10.738, 1.1642) (10.7532, 1.1556) (10.7684, 1.147) (10.7836, 1.1383) (10.7988, 1.1296) (10.8141, 1.1208) (10.8293, 1.1119) (10.8446, 1.103) (10.8598, 1.094) (10.8751, 1.0849) (10.8904, 1.0758) (10.9057, 1.0666) (10.921, 1.0573) (10.9364, 1.048) (10.9517, 1.0386) (10.967, 1.0292) (10.9824, 1.0197) (10.9978, 1.0101) (11.0131, 1.0004) (11.0285, 0.9907) (11.0439, 0.981) (11.0593, 0.9711) (11.0747, 0.9612) (11.0902, 0.9513) (11.1056, 0.9413) (11.121, 0.9312) (11.1365, 0.921) (11.1519, 0.9108) (11.1674, 0.9005) (11.1828, 0.8902) (11.1983, 0.8798) (11.2138, 0.8693) (11.2292, 0.8588) (11.2447, 0.8482) (11.2602, 0.8375) (11.2757, 0.8268) (11.2912, 0.816) (11.3036, 0.8073) (11.3129, 0.8008) (11.3191, 0.7964) (11.3222, 0.7942) knots 0 0 0 0 0 0 0.00416667 0.00833333 0.0125 0.01666667 0.02083333 0.025 0.02916667 0.03333333 0.0375 0.04166667 0.04583333 0.05 0.05416667 0.05833333 0.0625 0.06666667 0.07083333 0.075 0.07916667 0.08333333 0.0875 0.09166667 0.09583333 0.1 0.10416667 0.10833333 0.1125 0.11666667 0.12083333 0.125 0.12916667 0.13333333 0.1375 0.14166667 0.14583333 0.15 0.15416667 0.15833333 0.1625 0.16666667 0.17083333 0.175 0.17916667 0.18333333 0.1875 0.19166667 0.19583333 0.2 0.20416667 0.20833333 0.2125 0.21666667 0.22083333 0.225 0.22916667 0.23333333 0.2375 0.24166667 0.24583333 0.25 0.25416667 0.25833333 0.2625 0.26666667 0.27083333 0.275 0.27916667 0.28333333 0.2875 0.29166667 0.29583333 0.3 0.30416667 0.30833333 0.3125 0.31666667 0.32083333 0.325 0.32916667 0.33333333 0.3375 0.34166667 0.34583333 0.35 0.35416667 0.35833333 0.3625 0.36666667 0.37083333 0.375 0.37916667 0.38333333 0.3875 0.39166667 0.39583333 0.4 0.40416667 0.40833333 0.4125 0.41666667 0.42083333 0.425 0.42916667 0.43333333 0.4375 0.44166667 0.44583333 0.45 0.45416667 0.45833333 0.4625 0.46666667 0.47083333 0.475 0.47916667 0.48333333 0.4875 0.49166667 0.49583333 0.5 0.50416667 0.50833333 0.5125 0.51666667 0.52083333 0.525 0.52916667 0.53333333 0.5375 0.54166667 0.54583333 0.55 0.55416667 0.55833333 0.5625 0.56666667 0.57083333 0.575 0.57916667 0.58333333 0.5875 0.59166667 0.59583333 0.6 0.60416667 0.60833333 0.6125 0.61666667 0.62083333 0.625 0.62916667 0.63333333 0.6375 0.64166667 0.64583333 0.65 0.65416667 0.65833333 0.6625 0.66666667 0.67083333 0.675 0.67916667 0.68333333 0.6875 0.69166667 0.69583333 0.7 0.70416667 0.70833333 0.7125 0.71666667 0.72083333 0.725 0.72916667 0.73333333 0.7375 0.74166667 0.74583333 0.75 0.75416667 0.75833333 0.7625 0.76666667 0.77083333 0.775 0.77916667 0.78333333 0.7875 0.79166667 0.79583333 0.8 0.80416667 0.80833333 0.8125 0.81666667 0.82083333 0.825 0.82916667 0.83333333 0.8375 0.84166667 0.84583333 0.85 0.85416667 0.85833333 0.8625 0.86666667 0.87083333 0.875 0.87916667 0.88333333 0.8875 0.89166667 0.89583333 0.9 0.90416667 0.90833333 0.9125 0.91666667 0.92083333 0.925 0.92916667 0.93333333 0.9375 0.94166667 0.94583333 0.95 0.95416667 0.95833333 0.9625 0.96666667 0.97083333 0.975 0.97916667 0.98333333 0.9875 0.99166667 0.99583333 1 1 1 1 1 1
  spline S2 degree 5 poles (8.6122, -1.7628) (8.6123, -1.7628) (8.6124, -1.7628) (8.6125, -1.7628) (8.6127, -1.7629) (8.6129, -1.7629) (8.6131, -1.763) (8.6133, -1.763) (8.6134, -1.763) (8.6134, -1.763) knots 0 0 0 0 0 0 0.2 0.4 0.6 0.8 1 1 1 1 1 1
  spline S3 degree 5 poles (8.6122, 1.7628) (8.6123, 1.7628) (8.6124, 1.7628) (8.6125, 1.7628) (8.6127, 1.7629) (8.6129, 1.7629) (8.6131, 1.763) (8.6133, 1.763) (8.6134, 1.763) (8.6134, 1.763) knots 0 0 0 0 0 0 0.2 0.4 0.6 0.8 1 1 1 1 1 1
  line L0 (0, 0) -> (8.6122, -1.7628)
  line L1 (0, 0) -> (8.6122, 1.7628)
  arc A0 (11.3222, -0.7942) -> (11.3222, 0.7942) centre (0, 0) ccw
  point P0 (8.617, -1.7636)
  point P1 (8.6231, -1.7646)
  point P2 (8.6315, -1.7658)
  point P3 (8.6424, -1.7672)
  point P4 (8.6558, -1.7687)
  point P5 (8.6716, -1.7702)
  point P6 (8.6898, -1.7716)
  point P7 (8.7106, -1.7728)
  point P8 (8.7337, -1.7738)
  point P9 (8.7594, -1.7745)
  point P10 (8.7875, -1.7748)
  point P11 (8.818, -1.7746)
  point P12 (8.8509, -1.7738)
  point P13 (8.8863, -1.7724)
  point P14 (8.9241, -1.7703)
  point P15 (8.9643, -1.7673)
  point P16 (9.0069, -1.7635)
  point P17 (9.0518, -1.7587)
  point P18 (9.099, -1.7529)
  point P19 (9.1486, -1.7459)
  point P20 (9.2005, -1.7377)
  point P21 (9.2546, -1.7282)
  point P22 (9.311, -1.7174)
  point P23 (9.3695, -1.7051)
  point P24 (9.4302, -1.6913)
  point P25 (9.4931, -1.676)
  point P26 (9.5581, -1.6589)
  point P27 (9.6251, -1.6402)
  point P28 (9.6941, -1.6196)
  point P29 (9.7651, -1.5971)
  point P30 (9.8381, -1.5727)
  point P31 (9.9129, -1.5462)
  point P32 (9.9896, -1.5176)
  point P33 (10.068, -1.4869)
  point P34 (10.1482, -1.454)
  point P35 (10.2301, -1.4187)
  point P36 (10.3136, -1.3811)
  point P37 (10.3987, -1.3411)
  point P38 (10.4852, -1.2986)
  point P39 (10.5733, -1.2535)
  point P40 (10.6627, -1.2058)
  point P41 (10.7535, -1.1555)
  point P42 (10.8455, -1.1024)
  point P43 (10.9387, -1.0465)
  point P44 (11.0331, -0.9879)
  point P45 (11.1285, -0.9263)
  point P46 (11.2249, -0.8617)
  point P47 (8.617, 1.7636)
  point P48 (8.6231, 1.7646)
  point P49 (8.6315, 1.7658)
  point P50 (8.6424, 1.7672)
  point P51 (8.6558, 1.7687)
  point P52 (8.6716, 1.7702)
  point P53 (8.6898, 1.7716)
  point P54 (8.7106, 1.7728)
  point P55 (8.7337, 1.7738)
  point P56 (8.7594, 1.7745)
  point P57 (8.7875, 1.7748)
  point P58 (8.818, 1.7746)
  point P59 (8.8509, 1.7738)
  point P60 (8.8863, 1.7724)
  point P61 (8.9241, 1.7703)
  point P62 (8.9643, 1.7673)
  point P63 (9.0069, 1.7635)
  point P64 (9.0518, 1.7587)
  point P65 (9.099, 1.7529)
  point P66 (9.1486, 1.7459)
  point P67 (9.2005, 1.7377)
  point P68 (9.2546, 1.7282)
  point P69 (9.311, 1.7174)
  point P70 (9.3695, 1.7051)
  point P71 (9.4302, 1.6913)
  point P72 (9.4931, 1.676)
  point P73 (9.5581, 1.6589)
  point P74 (9.6251, 1.6402)
  point P75 (9.6941, 1.6196)
  point P76 (9.7651, 1.5971)
  point P77 (9.8381, 1.5727)
  point P78 (9.9129, 1.5462)
  point P79 (9.9896, 1.5176)
  point P80 (10.068, 1.4869)
  point P81 (10.1482, 1.454)
  point P82 (10.2301, 1.4187)
  point P83 (10.3136, 1.3811)
  point P84 (10.3987, 1.3411)
  point P85 (10.4852, 1.2986)
  point P86 (10.5733, 1.2535)
  point P87 (10.6627, 1.2058)
  point P88 (10.7535, 1.1555)
  point P89 (10.8455, 1.1024)
  point P90 (10.9387, 1.0465)
  point P91 (11.0331, 0.9879)
  point P92 (11.1285, 0.9263)
  point P93 (11.2249, 0.8617)
sketch "Sketch2" plane through (0, 0, 0) normal (0, 0, 1) x (1, 0, 0) in component "Component"
  circle A0 centre (0, 0) radius 6.2425
extrude "Extrude1" add sketch "Sketch2" along normal blind 6 makes body 1 in component "Component"
extrude "Extrude2" add sketch "Sketch1 (2)" along normal blind 6 separate body makes body 2 in component "Component"
pattern_circular "C-Pattern1" count 8 over 360 about axis through (0, 0, 1.75) along (0, 0, 1) of "Extrude2" makes body 3 at (3.2293, 4.8915, 4) makes body 4 at (0.5877, 2.8711, 4) makes body 5 at (-1.6147, 2.4457, 2) makes body 6 at (-2.8711, -0.5877, 2) makes body 7 at (-2.4457, -1.6147, 2) makes body 8 at (-0.5877, -2.8711, 2) makes body 9 at (4.8915, -3.2293, 4) in component "Component"
combine "Combine1" operation add target body 1 tool bodies 2 3 4 5 6 7 8 9 in component "Component"
sketch "Sketch3" plane through (0, 0, 0) normal (0, 0, 1) x (1, 0, 0) in component "Component"
  line L0 (0, 0) -> (48.2549, 0) construction
  line L1 (48.2549, 0) -> (48.2549, 3) construction
  line L2 (48.2549, 3) -> (0, 3) construction
  line L3 (0, 3) -> (0, 0) construction
  constraint perpendicular L0 L1
  constraint parallel L0 L2
  constraint parallel L1 L3
extrude "Extrude3" cut sketch "Sketch1" against normal blind 6 contours A16 bodies 1 in component "Component"
component "Component" placed x (1, 0, 0) y (0, 1, 0) z (0, 0, 1) at (0, 0, 0)
component "Component" placed x (1, 0, 0) y (0, 1, 0) z (0, 0, 1) at (25, 0, 0)

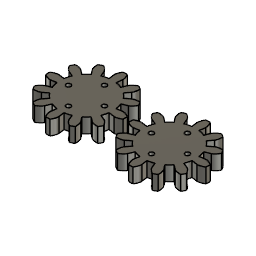
design "card-shuffler-driver-gears"
part number: 2026-07-29-20-33-23-439
part number: 2026-07-29-23-12-29-197
Autodesk Fusion 360 part; units mm, degrees